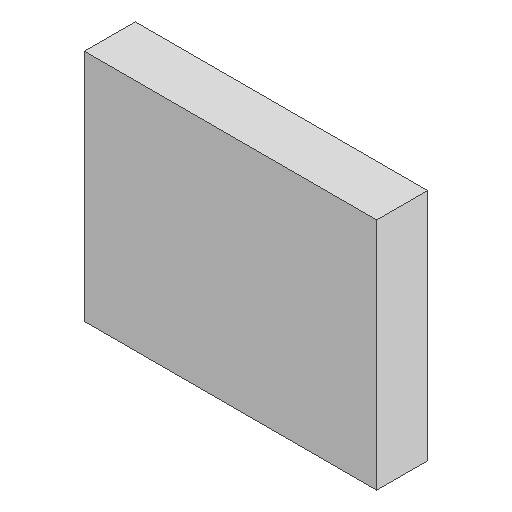
# Autodesk Inventor part: XP2ScaleModel
Saved by Autodesk Inventor 2026.2 (Build 302298000, 298)
## iProperties
Created: 2026-03-31
Part Number: XP2ScaleModel
Material: Generic
Document SubType Name: Modeling
Designer: gaoet
Density: 1 g/cm^3
Appearance: Default
Author: gaoet
Autodesk Inventor part; units mm, degrees
ref_plane "YZ Plane" through (0, 0, 0) normal (1, 0, 0) x (0, 1, 0)
ref_plane "XZ Plane" through (0, 0, 0) normal (0, 1, 0) x (-1, 0, 0)
ref_plane "XY Plane" through (0, 0, 0) normal (0, 0, 1) x (1, 0, 0)
sketch "Sketch1" plane through (0, 0, 0) normal (0, 0, 1) x (1, 0, 0)
  line L0 (-158, -126.5) -> (158, -126.5)
  line L1 (158, -126.5) -> (158, 126.5)
  line L2 (158, 126.5) -> (-158, 126.5)
  line L3 (-158, 126.5) -> (-158, -126.5)
  line L4 (-158, -126.5) -> (158, 126.5) construction
  line L5 (158, -126.5) -> (-158, 126.5) construction
  point P0 (0, 0)
  dimension "d0" = 316
  dimension "d1" = 253
  constraints: 12 end point, 2 midpoint, 2 parallel, 1 horizontal, 1 perpendicular
  measures "d0" distance of L2.end L1.end
  measures "d1" distance of L0.end L1.end
extrude "Extrusion1" add sketch "Sketch1" along normal blind 55
body "Solid1"
